Autodesk Fusion 360 part; units mm, degrees
(part 15 of 15)
component "Base2" placed x (0.999769, 0, -0.021505) y (0, 1, 0) z (0.021505, 0, 0.999769) at (96.4053, 130.8893, 48.2321)
component "Spur Gear 22 teeth" placed x (-0.991961, 0, -0.126542) y (0.126542, 0, -0.991961) z (0, -1, 0) at (35, 525, -35) in component "Component'"
component "Spur Gear 22 teeth" placed x (0.967075, 0, 0.254492) y (-0.254492, 0, 0.967075) z (0, -1, 0) at (-35, 525, -35) in component "Component'"
component "Spur Gear 22 teeth" placed x (-0.588525, 0, 0.808479) y (-0.808479, 0, -0.588525) z (0, -1, 0) at (-35, 525, 35) in component "Component'"
component "Spur Gear 22 teeth" placed x (-0.209976, 0, 0.977707) y (-0.977707, 0, -0.209976) z (0, -1, 0) at (35, 525, 35) in component "Component'"
component "Spur Gear 28 teeth" placed x (-0.786213, 0, 0.617955) y (-0.617955, 0, -0.786213) z (0, -1, 0) at (0, 240, 0) in component "SUN  gear"
